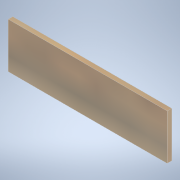
# Autodesk Inventor part: Eyebrow2
Saved by Autodesk Inventor 2021 (Build 250183000, 183)
## iProperties
Created: 2023-05-31
Part Number: Eyebrow2
Material: Wood (Maple)
Document SubType Name: Modeling
Designer: shrus
Density: 0.67 g/cm^3
Appearance: Natural Maple - Glossy Dark Tint
Author: shrus
Autodesk Inventor part; units mm, degrees
ref_plane "YZ Plane" through (0, 0, 0) normal (1, 0, 0) x (0, 1, 0)
ref_plane "XZ Plane" through (0, 0, 0) normal (0, 1, 0) x (-1, 0, 0)
ref_plane "XY Plane" through (0, 0, 0) normal (0, 0, 1) x (1, 0, 0)
sketch "Sketch1" plane through (0, 0, 0) normal (0, 0, 1) x (1, 0, 0)
  line L0 (-12.6223, 11.5839) -> (22.3777, 11.5839)
  line L1 (22.3777, 11.5839) -> (22.3777, 1.5839)
  line L2 (22.3777, 1.5839) -> (-12.6223, 1.5839)
  line L3 (-12.6223, 1.5839) -> (-12.6223, 11.5839)
  point P0 (0, 0)
  dimension "d0" = 35
  dimension "d1" = 10
  constraints: 8 end point, 3 perpendicular, 1 horizontal
  measures "d0" distance of L0.start L0.end
  measures "d1" distance of L0.end L1.end
extrude "Extrusion1" add sketch "Sketch1" along normal blind 1
body "Solid1"
